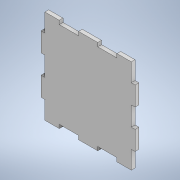
# Autodesk Inventor part: Rightandleft_2
Saved by Autodesk Inventor 2020 (Build 240168000, 168)
## iProperties
Created: 2020-12-28
Part Number: Rightandleft_2
Material: Generic
Document SubType Name: Modeling
Designer: solar
Density: 1 g/cm^3
Appearance: Default
Author: solar
Autodesk Inventor part; units mm, degrees
ref_plane "YZ Plane" through (0, 0, 0) normal (1, 0, 0) x (0, 1, 0)
ref_plane "XZ Plane" through (0, 0, 0) normal (0, 1, 0) x (-1, 0, 0)
ref_plane "XY Plane" through (0, 0, 0) normal (0, 0, 1) x (1, 0, 0)
sketch "Sketch1" plane through (0, 0, 0) normal (0, 0, 1) x (1, 0, 0)
  line L0 (-69, -75) -> (-46.125, -75)
  line L1 (-46.125, -69) -> (-46.125, -75)
  line L2 (-15.375, -69) -> (-46.125, -69)
  line L3 (-15.375, -75) -> (-15.375, -69)
  line L4 (-46.125, 69) -> (-46.125, 75)
  line L5 (-15.375, 69) -> (-46.125, 69)
  line L6 (-15.375, 75) -> (-15.375, 69)
  line L7 (-75, -15.375) -> (-69, -15.375)
  line L8 (-69, -46.125) -> (-75, -46.125)
  line L9 (-69, 46.125) -> (-75, 46.125)
  line L10 (-75, 15.375) -> (-69, 15.375)
  line L11 (0, -75) -> (-15.375, -75)
  line L12 (-46.125, -75) -> (-69, -75)
  line L13 (-69, 75) -> (-46.125, 75)
  line L14 (-15.375, 75) -> (0, 75)
  line L15 (-69, 46.125) -> (-69, 75)
  line L16 (-75, 46.125) -> (-75, 15.375)
  line L17 (-69, 15.375) -> (-69, -15.375)
  line L18 (-75, -15.375) -> (-75, -46.125)
  line L19 (-69, -46.125) -> (-69, -75)
  line L20 (0, 0) -> (0, 15.375)
  line L21 (0, 75) -> (0, -75)
  line L22 (69, -75) -> (46.125, -75)
  line L23 (46.125, -69) -> (46.125, -75)
  line L24 (15.375, -69) -> (46.125, -69)
  line L25 (15.375, -75) -> (15.375, -69)
  line L26 (46.125, 69) -> (46.125, 75)
  line L27 (15.375, 69) -> (46.125, 69)
  line L28 (15.375, 75) -> (15.375, 69)
  line L29 (75, -15.375) -> (69, -15.375)
  line L30 (69, -46.125) -> (75, -46.125)
  line L31 (69, 46.125) -> (75, 46.125)
  line L32 (75, 15.375) -> (69, 15.375)
  line L33 (0, -75) -> (15.375, -75)
  line L34 (46.125, -75) -> (69, -75)
  line L35 (69, 75) -> (46.125, 75)
  line L36 (15.375, 75) -> (0, 75)
  line L37 (69, 46.125) -> (69, 75)
  line L38 (75, 46.125) -> (75, 15.375)
  line L39 (69, 15.375) -> (69, -15.375)
  line L40 (75, -15.375) -> (75, -46.125)
  line L41 (69, -46.125) -> (69, -75)
  constraints: 84 end point, 18 symmetric about line, 3 perpendicular, 2 parallel, 2 vertical, 1 horizontal
extrude "Extrusion1" add sketch "Sketch1" along normal blind 6
body "Solid1"
